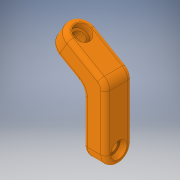
# Autodesk Inventor part: Link2
Saved by Autodesk Inventor 2019 (Build 230136000, 136)
## iProperties
Created: 2022-07-14
Part Number: Link2
Material: Generic
Document SubType Name: Modeling
Designer: zreik
Density: 1 g/cm^3
Appearance: Orange
d46: 10.000 mm
Author: zreik
Autodesk Inventor part; units mm, degrees
ref_plane "YZ Plane" through (0, 0, 0) normal (1, 0, 0) x (0, 1, 0)
sketch "Sketch1" plane through (0, 0, 0) normal (0, 0, 1) x (1, 0, 0)
  line L0 (37.7128, 0) -> (0, 0)
  line L1 (0, 0) -> (34.8308, 60.3287)
  line L2 (27.7128, 0) -> (27.7128, 19.1132)
  line L3 (25.2128, 23.4434) -> (16.4545, 28.5)
  line L4 (37.7128, 0) -> (37.7128, 24.8868)
  line L5 (35.2128, 29.2169) -> (21.4545, 37.1603)
  arc A0 (27.7128, 19.1132) -> (25.2128, 23.4434) centre (22.7128, 19.1132) ccw
  arc A1 (37.7128, 24.8868) -> (35.2128, 29.2169) centre (32.7128, 24.8868) ccw
  line L6 (21.4545, 37.1603) -> (16.4545, 28.5)
  line L7 (21.4545, 37.1603) -> (35.2128, 29.2169)
  line L8 (16.4545, 28.5) -> (25.2128, 23.4434)
  line L9 (27.7128, 0) -> (37.7128, 0)
  line L10 (37.7128, 0) -> (37.7128, 24.8868)
  line L11 (27.7128, 0) -> (37.7128, 0)
  line L12 (37.7128, 0) -> (37.7128, 24.8868)
  line L13 (35.2128, 29.2169) -> (21.4545, 37.1603)
  line L14 (21.4545, 37.1603) -> (16.4545, 28.5)
  line L15 (16.4545, 28.5) -> (25.2128, 23.4434)
  line L16 (27.7128, 19.1132) -> (27.7128, 0)
  point P0 (25, 43.3013)
  point P1 (27.7128, 22)
  dimension "d37" = 60
  dimension "d38" = 10
  dimension "d39" = 10
  dimension "d40" = 0
  dimension "d41" = 0
  dimension "d42" = 22
  dimension "d43" = 13
  dimension "d44" = 120
  dimension "d45" = 5
  constraints: 34 end point, 9 collinear, 6 point on line, 4 point on circle, 4 tangent, 2 centre point, 2 parallel, 1 coincident, 1 equal radius, 1 horizontal, 1 vertical
  measures "d37" angle of L1 L0
  measures "d38" distance between parallel lines of L3 L5
  measures "d39" distance between parallel lines of L4 L2
  measures "d40" distance from line of L1 L3.end
  measures "d41" distance from line of L1 L5.end
  measures "d42" distance of L2.start point (27.713, 22)
  measures "d43" distance of point (27.713, 22) L3.end
  measures "d44" angle of L2 L3
  measures "d45" radius of A0
extrude "Extrusion1" add sketch "Sketch1" along normal blind 12 contours L0 L2 A0 L3 L1 L5 A1 L4
ref_plane "Work Plane1" through (35.2128, 29.2169, 0) normal (0.5, 0.8660254, 0) x (-0.8660254, 0.5, 0)
sketch "Sketch2" plane through (35.2128, 29.2169, 0) normal (0.5, 0.8660254, 0) x (-0.8660254, 0.5, 0)
  circle A0 centre (15.8868, 6) radius 6
  line L0 (15.8868, 0) -> (15.8868, 12) projected
  line L1 (0, 12) -> (15.8868, 12) projected
  dimension "d5" = 12
  dimension "d47" = 0
  dimension "d48" = 6
  constraints: 1 centre point
  measures "d5" diameter of A0
  measures "d47" distance from line of L0 A0.centre
  measures "d48" distance from line of L1 A0.centre
extrude "Extrusion2" add sketch "Sketch2" against normal blind 10
ref_plane "Work Plane2" through (37.7128, 24.8868, 0) normal (1, 0, 0) x (0, 1, 0)
sketch "Sketch3" plane through (37.7128, 24.8868, 0) normal (1, 0, 0) x (0, 1, 0)
  circle A0 centre (-24.8868, 6) radius 6
  line L0 (-24.8868, 0) -> (-24.8868, 12) projected
  line L1 (-24.8868, 0) -> (0, 0) projected
  point P0 (43.3013, 10)
  point P1 (3.6132, 12)
  dimension "d10" = 12
  dimension "d49" = 0
  dimension "d50" = 6
  constraints: 1 centre point, 1 other
  measures "d10" diameter of A0
  measures "d49" distance from line of L0 A0.centre
  measures "d50" distance from line of L1 A0.centre
extrude "Extrusion3" add sketch "Sketch3" against normal blind 10
sketch "Sketch4" plane through (30.2128, 20.5566, 0) normal (-0.5, -0.8660254, 0) x (0.8660254, -0.5, 0)
  circle A0 centre (-15.8868, 6) radius 2.5
  circle A1 centre (-15.8868, 6) radius 6 projected
  point P0 (-15.8868, 0)
  point P1 (-15.8868, 12)
  dimension "d15" = 5
  constraints: 1 centre point, 1 concentric
  measures "d15" diameter of A0
extrude "Extrusion4" cut sketch "Sketch4" along normal through all both and the other way through all contours A0
sketch "Sketch5" plane through (27.7128, 24.8868, 0) normal (-1, 0, 0) x (0, 0, 1)
  circle A0 centre (6, -24.8868) radius 2.5
  arc A1 (0, -24.8868) -> (12, -24.8868) centre (6, -24.8868) ccw projected
  dimension "d18" = 5
  constraints: 1 centre point, 1 concentric
  measures "d18" diameter of A0
extrude "Extrusion5" cut sketch "Sketch5" along normal through all both and the other way through all
sketch "Sketch6" plane through (35.2128, 29.2169, 0) normal (0.5, 0.8660254, 0) x (0.8660254, -0.5, 0)
  circle A0 centre (-15.8868, -6) radius 3.6
  circle A1 centre (-15.8868, -6) radius 2.5
  arc A2 (-15.8868, 0) -> (-15.8868, 0) centre (-15.8868, -6) ccw projected
  point P0 (0, -10)
  dimension "d21" = 5
  dimension "d22" = 7.2
  constraints: 2 centre point, 1 coincident, 2 other
  measures "d21" diameter of A1
  measures "d22" diameter of A0
extrude "Extrusion6" cut sketch "Sketch6" against normal blind 3 contours A0
sketch "Sketch7" plane through (30.2128, 20.5566, 0) normal (-0.5, -0.8660254, 0) x (0.8660254, -0.5, 0)
  circle A0 centre (-15.8868, 6) radius 3.6
  circle A1 centre (-15.8868, 6) radius 2.5
  arc A2 (-13.3868, 6) -> (-13.3868, 6) centre (-15.8868, 6) ccw projected
  point P0 (-15.8868, 0)
  dimension "d25" = 5
  dimension "d26" = 7.2
  constraints: 2 centre point, 1 coincident, 1 concentric
  measures "d25" diameter of A1
  measures "d26" diameter of A0
extrude "Extrusion7" cut sketch "Sketch7" along normal mid plane 6
sketch "Sketch8" plane through (27.7128, 24.8868, 0) normal (-1, 0, 0) x (0, 0, 1)
  circle A0 centre (6, -24.8868) radius 3.6
  circle A1 centre (6, -24.8868) radius 2.5
  arc A2 (8.5, -24.8868) -> (8.5, -24.8868) centre (6, -24.8868) ccw projected
  point P0 (0, -24.8868)
  dimension "d29" = 7.2
  dimension "d30" = 5
  constraints: 2 centre point, 1 coincident, 1 concentric
  measures "d29" diameter of A0
  measures "d30" diameter of A1
extrude "Extrusion8" cut sketch "Sketch8" along normal mid plane 6
sketch "Sketch9" plane through (37.7128, 24.8868, 0) normal (1, 0, 0) x (0, 0, -1)
  circle A0 centre (-6, -24.8868) radius 3.6
  circle A1 centre (-6, -24.8868) radius 2.5
  circle A2 centre (-6, -24.8868) radius 2.5 projected
  point P0 (0, -24.8868)
  dimension "d33" = 5
  dimension "d34" = 7.2
  constraints: 2 centre point, 1 coincident, 1 concentric
  measures "d33" diameter of A1
  measures "d34" diameter of A0
extrude "Extrusion9" cut sketch "Sketch9" against normal blind 3
fillet "Fillet1" radius 2 16 edges at (16.2583, 40.1603, 6) (28.3336, 33.1886, 0) (37.0429, 27.3868, 0) (37.7128, 12.4434, 0) (37.7128, -6, 6) (37.7128, 12.4434, 12) (37.0429, 27.3868, 12) (28.3336, 33.1886, 12) (27.0429, 21.6132, 12) (27.7128, 9.5566, 12) (27.7128, -6, 6) (27.7128, 9.5566, 0) (27.0429, 21.6132, 0) (20.8336, 25.9717, 0) (11.2583, 31.5, 6) (20.8336, 25.9717, 12)
equation "\"d38\" = d46"
equation "\"d39\" = d46"
equation "\"d3\" = width"
equation "\"d5\" = width"
equation "\"d48\" = 0.5 * width"
equation "\"d8\" = thickness"
equation "\"d10\" = width"
equation "\"d50\" = 0.5 * width"
equation "\"d13\" = thickness"
equation "\"thickness\" = thickness_1"
equation "\"width\" = width_1"
equation "\"d46\" = 10"
equation "\"thickness_1\" = 10"
equation "\"width_1\" = 12"
body "Solid1"
